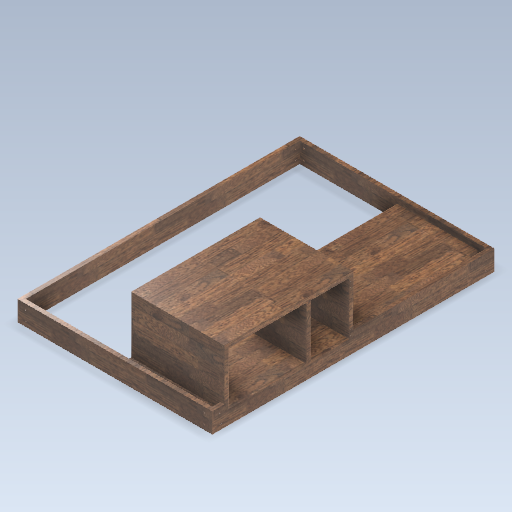
# Autodesk Inventor part: Middle Floor
Saved by Autodesk Inventor 2020 (Build 240168000, 168)
## iProperties
Created: 2020-06-26
Part Number: Middle Floor
Material: Generic
Document SubType Name: Modeling
Designer: Abbas
Density: 1 g/cm^3
Appearance: Default
Author: Abbas
Autodesk Inventor part; units mm, degrees
sketch "Sketch1" plane through (0, 0, 0) normal (0, 1, 0) x (-1, 0, 0)
  line L0 (478.912, 694) -> (-478.912, 694)
  line L1 (-478.912, 694) -> (-478.912, -694)
  line L2 (-478.912, -694) -> (478.912, -694)
  line L3 (478.912, -694) -> (478.912, 694)
  line L4 (478.912, 694) -> (-478.912, -694) construction
  line L5 (-478.912, 694) -> (478.912, -694) construction
  line L6 (458.912, 674) -> (-458.912, 674)
  line L7 (-458.912, 674) -> (-458.912, -674)
  line L8 (-458.912, -674) -> (458.912, -674)
  line L9 (458.912, -674) -> (458.912, 674)
  line L10 (458.912, 674) -> (-458.912, -674) construction
  line L11 (-458.912, 674) -> (458.912, -674) construction
  line L12 (-458.912, 400) -> (-438.912, 400)
  line L13 (-438.912, 400) -> (-438.912, -400)
  line L14 (-438.912, -400) -> (-458.912, -400)
  line L15 (-458.912, -400) -> (-458.912, 400)
  line L16 (-458.912, 400) -> (-438.912, -400) construction
  line L17 (-438.912, 400) -> (-458.912, -400) construction
  line L18 (-20, -654) -> (-350, -654)
  line L19 (-350, -654) -> (-350, -674)
  line L20 (-350, -674) -> (350, -674)
  line L21 (0, -664) -> (-0.1429, -664.0041) construction
  line L22 (-0.1428, -663.9959) -> (0, -664) construction
  line L23 (0, -654) -> (0, -674)
  line L24 (-20, 654) -> (-350, 654)
  line L25 (-350, 654) -> (-350, 674)
  line L26 (0, -654) -> (0, 674)
  line L27 (0, 674) -> (-20, 674)
  line L28 (-20, 674) -> (-20, -674)
  point P0 (0, 0)
  point P1 (-448.912, 0)
  point P2 (-458.912, 0)
  point P3 (0, 654)
  dimension "d0" = 957.824
  dimension "d1" = 1388
  dimension "d2" = 917.824
  dimension "d3" = 1348
  dimension "d6" = 20
  dimension "d7" = 800
  dimension "d11" = 20
  dimension "d96" = 20
  dimension "d97" = 90
  constraints: 58 end point, 10 midpoint, 7 parallel, 5 point on line, 4 horizontal, 4 perpendicular, 2 collinear, 1 vertical
  measures "d0" distance of L2.end L1.end
  measures "d1" distance of L1.end L0.end
  measures "d2" distance of L8.end L7.end
  measures "d3" distance of L7.end L6.end
  measures "d6" distance of L13.end L14.end
  measures "d7" distance of L12.end L13.end
  measures "d11" distance of L19.end L18.end
  measures "d96" distance of L26.end L27.end
  measures "d97" angle of L28 L27
extrude "Extrusion7" add sketch "Sketch1" along normal blind 100
sketch "Sketch2" plane through (478.912, 0, 694) normal (1, 0, 0) x (0, 0, -1)
  line L0 (0, 0) -> (0, 100) projected
  line L1 (0, 100) -> (1388, 100) projected
  point P0 (694, 0)
  point P1 (40, 75)
  dimension "d40" = 40
  dimension "d41" = 25
  measures "d40" distance from line of L0 point (40, 75)
  measures "d41" distance from line of L1 point (40, 75)
hole "Hole1" at (478.912, 75, 654) direction (-1, 0, 0) diameter 8 end through all
sketch "Sketch3" plane through (478.912, 0, 694) normal (1, 0, 0) x (0, 0, -1)
  line L0 (0, 0) -> (0, 100) projected
  line L1 (0, 0) -> (1388, 0) projected
  point P0 (694, 0)
  point P1 (40, 25)
  dimension "d42" = 40
  dimension "d43" = 25
  measures "d42" distance from line of L0 point (40, 25)
  measures "d43" distance from line of L1 point (40, 25)
hole "Hole2" at (478.912, 25, 654) direction (-1, 0, 0) diameter 8 end through all
sketch "Sketch4" plane through (478.912, 0, 694) normal (1, 0, 0) x (0, 0, -1)
  line L0 (1388, 0) -> (1388, 100) projected
  line L1 (0, 100) -> (1388, 100) projected
  point P0 (694, 0)
  point P1 (1348, 75)
  dimension "d58" = 40
  dimension "d59" = 25
  measures "d58" distance from line of L0 point (1348, 75)
  measures "d59" distance from line of L1 point (1348, 75)
hole "Hole3" at (478.912, 75, -654) direction (-1, 0, 0) diameter 8 end through all
sketch "Sketch5" plane through (478.912, 0, 694) normal (1, 0, 0) x (0, 0, -1)
  line L0 (1388, 0) -> (1388, 100) projected
  line L1 (0, 0) -> (1388, 0) projected
  point P0 (694, 0)
  point P1 (1348, 25)
  dimension "d60" = 40
  dimension "d61" = 25
  measures "d60" distance from line of L0 point (1348, 25)
  measures "d61" distance from line of L1 point (1348, 25)
hole "Hole4" at (478.912, 25, -654) direction (-1, 0, 0) diameter 8 end through all
sketch "Sketch6" plane through (-478.912, 0, 694) normal (0, 0, 1) x (1, 0, 0)
  line L0 (0, 100) -> (957.824, 100) projected
  line L1 (957.824, 0) -> (957.824, 100) projected
  line L2 (0, 0) -> (957.824, 0) projected
  point P0 (478.912, 0)
  point P1 (917.824, 75)
  point P2 (917.824, 25)
  dimension "d69" = 25
  dimension "d70" = 40
  dimension "d71" = 40
  dimension "d72" = 25
  measures "d69" distance from line of L0 point (917.824, 75)
  measures "d70" distance from line of L1 point (917.824, 75)
  measures "d71" distance from line of L1 point (917.824, 25)
  measures "d72" distance from line of L2 point (917.824, 25)
hole "Hole5" at (438.912, 75, 694) at (438.912, 25, 694) direction (0, 0, -1) diameter 8 end through all
sketch "Sketch7" plane through (-478.912, 0, 694) normal (0, 0, 1) x (1, 0, 0)
  line L0 (0, 0) -> (0, 100) projected
  line L1 (0, 100) -> (957.824, 100) projected
  point P0 (478.912, 0)
  point P1 (40, 75)
  dimension "d87" = 40
  dimension "d88" = 25
  measures "d87" distance from line of L0 point (40, 75)
  measures "d88" distance from line of L1 point (40, 75)
hole "Hole6" at (-438.912, 75, 694) direction (0, 0, -1) diameter 8 end through all
sketch "Sketch8" plane through (-478.912, 0, 694) normal (0, 0, 1) x (1, 0, 0)
  line L0 (0, 0) -> (0, 100) projected
  line L1 (0, 0) -> (957.824, 0) projected
  point P0 (478.912, 0)
  point P1 (40, 25)
  dimension "d89" = 40
  dimension "d90" = 25
  measures "d89" distance from line of L0 point (40, 25)
  measures "d90" distance from line of L1 point (40, 25)
hole "Hole7" at (-438.912, 25, 694) direction (0, 0, -1) diameter 8 end through all
ref_plane "Work Plane1" through (-458.912, 100, 0) normal (0, 0, 1) x (1, 0, 0)
extrude "Extrusion10" add sketch "Sketch1" along normal blind 50 contours L28 L24 L25 L6 | L28 L8 L19 L18 | L12 L13 L14 L7
sketch "Sketch9" plane through (0, 50, 0) normal (0, 1, 0) x (1, 0, 0)
  line L0 (20, -674) -> (20, 674) projected
  line L1 (20, 674) -> (413.912, 674)
  line L2 (350, 674) -> (458.912, 674) projected
  line L3 (413.912, 674) -> (413.912, 629)
  line L4 (413.912, 629) -> (458.912, 629)
  line L5 (458.912, 674) -> (458.912, -674) projected
  line L6 (458.912, 629) -> (458.912, -629)
  line L7 (458.912, -629) -> (413.912, -629)
  line L8 (413.912, -629) -> (413.912, -674)
  line L9 (458.912, -674) -> (350, -674) projected
  line L10 (350, -674) -> (20, -674) projected
  line L11 (413.912, -674) -> (20, -674)
  line L12 (20, -674) -> (20, 674)
  point P0 (0, 0)
  dimension "d105" = 45
  dimension "d106" = 45
  dimension "d107" = 45
  dimension "d108" = 45
  constraints: 16 end point, 4 point on line, 3 perpendicular, 1 collinear, 1 horizontal, 1 vertical
  measures "d105" distance of L1.end L3.end
  measures "d106" distance of L3.end L4.end
  measures "d107" distance of L6.end L7.end
  measures "d108" distance of L7.end L8.end
extrude "Extrusion12" add sketch "Sketch9" along normal blind 20 contours L0 L1 L3 L4 L5 L7 L8 L9 L10
sketch "Sketch11" plane through (478.912, 0, 694) normal (1, 0, 0) x (0, 0, -1)
  line L0 (0, 100) -> (1388, 100) projected
  line L1 (0, 0) -> (0, 100) projected
  line L2 (0, 100) -> (1388, 100)
  line L3 (60, 100) -> (694, 100)
  line L4 (694, 100) -> (694, 70)
  line L5 (694, 70) -> (60, 70)
  line L6 (60, 70) -> (60, 100)
  line L7 (60, 100) -> (694, 70) construction
  line L8 (694, 100) -> (60, 70) construction
  point P0 (694, 0)
  point P1 (377, 85)
  point P2 (694, 100)
  dimension "d132" = 634
  dimension "d133" = 30
  dimension "d134" = 0
  dimension "d135" = 60
  constraints: 14 end point, 2 horizontal, 2 midpoint, 2 parallel, 1 perpendicular
  measures "d132" distance of L4.end L5.end
  measures "d133" distance of L3.end L4.end
  measures "d134" distance between parallel lines of L0 L3
  measures "d135" distance between parallel lines of L1 L6
extrude "Extrusion13" cut sketch "Sketch11" against normal blind 25
sketch "Sketch12" plane through (0, 70, 0) normal (0, 1, 0) x (1, 0, 0)
  line L0 (20, -634) -> (478.912, -634)
  line L1 (478.912, -634) -> (478.912, -614)
  line L2 (478.912, -614) -> (20, -614)
  line L3 (20, -614) -> (20, -634)
  line L4 (20, -634) -> (478.912, -614) construction
  line L5 (478.912, -634) -> (20, -614) construction
  line L6 (20, -20) -> (478.912, -20)
  line L7 (478.912, -20) -> (478.912, 0)
  line L8 (478.912, 0) -> (20, 0)
  line L9 (20, 0) -> (20, -20)
  line L10 (20, -20) -> (478.912, 0) construction
  line L11 (478.912, -20) -> (20, 0) construction
  line L12 (20, -230) -> (478.912, -230)
  line L13 (478.912, -230) -> (478.912, -210)
  line L14 (478.912, -210) -> (20, -210)
  line L15 (20, -210) -> (20, -230)
  line L16 (20, -230) -> (478.912, -210) construction
  line L17 (478.912, -230) -> (20, -210) construction
  line L18 (20, -210) -> (40, -210)
  line L19 (40, -210) -> (40, -20)
  line L20 (40, -20) -> (20, -20)
  line L21 (20, -20) -> (20, -210)
  line L22 (20, -210) -> (40, -20) construction
  line L23 (40, -210) -> (20, -20) construction
  line L24 (20, -614) -> (40, -614)
  line L25 (40, -614) -> (40, -230)
  line L26 (40, -230) -> (20, -230)
  line L27 (20, -230) -> (20, -614)
  line L28 (20, -614) -> (40, -230) construction
  line L29 (40, -614) -> (20, -230) construction
  point P0 (0, 0)
  point P1 (249.456, -624)
  point P2 (249.456, -10)
  point P3 (249.456, -220)
  point P4 (30, -115)
  point P5 (30, -422)
  dimension "d138" = 458.912
  dimension "d139" = 20
  dimension "d140" = 458.912
  dimension "d141" = 20
  dimension "d142" = 458.912
  dimension "d143" = 20
  dimension "d144" = 190
  dimension "d145" = 20
  dimension "d146" = 190
  dimension "d147" = 20
  dimension "d148" = 384
  constraints: 60 end point, 10 midpoint, 10 parallel, 5 horizontal, 5 perpendicular, 2 coincident
  measures "d138" distance of L2.end L1.end
  measures "d139" distance of L1.end L0.end
  measures "d140" distance of L8.end L7.end
  measures "d141" distance of L7.end L6.end
  measures "d142" distance of L14.end L13.end
  measures "d143" distance of L13.end L12.end
  measures "d144" distance between parallel lines of L14 L6
  measures "d145" distance of L6.start L19.end
  measures "d146" distance of L19.end L18.end
  measures "d147" distance of L12.start L25.end
  measures "d148" distance of L25.end L24.end
extrude "Extrusion14" add sketch "Sketch12" along normal blind 260
sketch "Sketch13" plane through (0, 330, 0) normal (0, 1, 0) x (1, 0, 0)
  line L0 (20, -634) -> (478.912, -634)
  line L1 (478.912, -634) -> (478.912, 0)
  line L2 (478.912, 0) -> (20, 0)
  line L3 (20, 0) -> (20, -634)
  line L4 (20, -634) -> (478.912, 0) construction
  line L5 (478.912, -634) -> (20, 0) construction
  point P0 (0, 0)
  point P1 (249.456, -317)
  dimension "d151" = 458.912
  dimension "d152" = 634
  constraints: 12 end point, 2 midpoint, 2 parallel, 1 coincident, 1 horizontal, 1 perpendicular
  measures "d151" distance of L2.end L1.end
  measures "d152" distance of L1.end L0.end
extrude "Extrusion15" add sketch "Sketch13" along normal blind 20
ref_plane "Work Plane2" through (0, 200, 0) normal (0, -1, 0) x (1, 0, 0)
ref_plane "Work Plane3" through (40, 70, 115) normal (0, 0, 1) x (1, 0, 0)
sketch "Sketch15" plane through (478.912, 0, 694) normal (1, 0, 0) x (0, 0, -1)
  circle A0 centre (681, 314.99) radius 1.875
  circle A1 centre (681, 289.19) radius 1.875
  circle A2 centre (681, 263.39) radius 1.875
  line L0 (674, 70) -> (674, 330) projected
  line L1 (674, 330) -> (694, 330)
  line L2 (694, 100) -> (694, 350) projected
  point P0 (694, 0)
  dimension "d166" = 3.75
  dimension "d167" = 3.75
  dimension "d168" = 3.75
  dimension "d169" = 15.01
  dimension "d170" = 25.8
  dimension "d171" = 25.8
  dimension "d172" = 13
  constraints: 3 centre point, 2 end point, 1 horizontal
  measures "d166" diameter of A0
  measures "d167" diameter of A1
  measures "d168" diameter of A2
  measures "d169" distance from line of L1 A0.centre
  measures "d170" distance of A0.centre A1.centre
  measures "d171" distance of A1.centre A2.centre
  measures "d172" distance from line of L2 A0.centre
extrude "Extrusion17" cut sketch "Sketch15" against normal blind 10
mirror "Mirror3" about plane through (0, 200, 0) normal (0, -1, 0) of "Extrusion17"
pattern_linear "Rectangular Pattern1" count 2 spacing 210 along (0, 0, 1) of "Extrusion17", "Mirror3"
body "Solid2"
